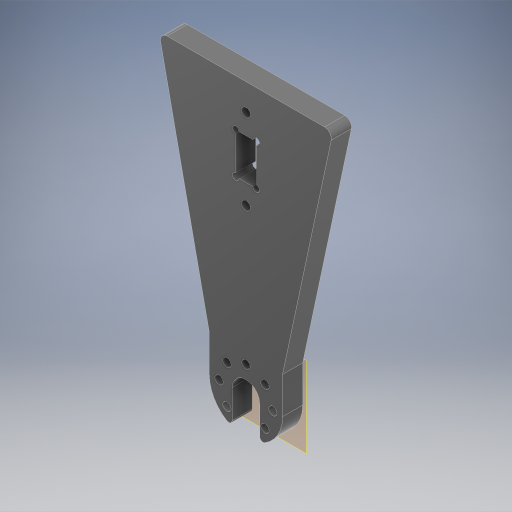
# Autodesk Inventor part: hand
Saved by Autodesk Inventor 2024 (Build 280153000, 153)
## iProperties
Created: 2024-09-04
Part Number: hand
Material: PMMA 플라스틱
Document SubType Name: Modeling
Designer: msi
Density: 1.188 g/cm^3
Appearance: 매끄러움 - 검은색
Mass: 19.7141 g
Surface Area: 78.213 cm^2
Volume: 16.5944 cm^3
Author: msi
Autodesk Inventor part; units mm, degrees
ref_plane "YZ Plane" through (0, 0, 0) normal (1, 0, 0) x (0, 1, 0)
ref_plane "XZ Plane" through (0, 0, 0) normal (0, 1, 0) x (-1, 0, 0)
ref_plane "XY Plane" through (0, 0, 0) normal (0, 0, 1) x (1, 0, 0)
ref_plane "작업 평면1" through (0, 0, 0) normal (0, 0, 1) x (1, 0, 0)
sketch "스케치1" plane through (0, 0, 0) normal (0, 0, 1) x (1, 0, 0)
  circle A0 centre (-5.6569, -5.6569) radius 1.2 projected
  circle A1 centre (5.6569, -5.6569) radius 1.2 projected
  circle A2 centre (5.6569, 5.6569) radius 1.2 projected
  circle A3 centre (-5.6569, 5.6569) radius 1.2 projected
  circle A4 centre (0, 0) radius 4 projected
  circle A5 centre (0, 0) radius 10.9 projected
  circle A6 centre (0, 8) radius 1.2 projected
  circle A7 centre (8, 0) radius 1.2 projected
  circle A8 centre (0, -8) radius 1.2 projected
  circle A9 centre (-8, 0) radius 1.2 projected
  line L0 (10.9, 0) -> (10.9, 10.9)
  line L1 (10.9, 10.9) -> (-10.9, 10.9)
  line L2 (-10.9, 10.9) -> (-10.9, 0)
  line L3 (-10.9, 10.9) -> (10.9, 10.9)
  line L4 (10.9, 80.9) -> (-10.9, 80.9)
  line L5 (10.9, 80.9) -> (25.9, 80.9)
  line L6 (25.9, 80.9) -> (10.9, 10.9)
  line L7 (-10.9, 80.9) -> (-25.9, 80.9)
  line L8 (-25.9, 80.9) -> (-10.9, 10.9)
  circle A10 centre (0, 72.9) radius 1.35
  circle A11 centre (0, 48.9) radius 1.35
  line L9 (-3.05, 54.85) -> (3.05, 54.85)
  line L10 (3.05, 54.85) -> (3.05, 66.95)
  line L11 (3.05, 66.95) -> (-3.05, 66.95)
  line L12 (-3.05, 66.95) -> (-3.05, 54.85)
  line L13 (-3.05, 54.85) -> (3.05, 66.95) construction
  line L14 (3.05, 54.85) -> (-3.05, 66.95) construction
  circle A12 centre (0, 0) radius 4.1
  circle A13 centre (5.6569, 5.6569) radius 1.25
  circle A14 centre (0, 8) radius 1.25
  circle A15 centre (-5.6569, 5.6569) radius 1.25
  circle A16 centre (-8, 0) radius 1.25
  circle A17 centre (-5.6569, -5.6569) radius 1.25
  circle A18 centre (0, -8) radius 1.25
  circle A19 centre (5.6569, -5.6569) radius 1.25
  circle A20 centre (8, 0) radius 1.25
  circle A21 centre (0, 0) radius 10.9
  line L15 (-4.1, 0) -> (-4.1, -10.0995)
  line L16 (4.1, 0) -> (4.1, -10.0995)
  point P0 (0, 0)
  point P1 (0, 60.9)
  dimension "d22" = 2.7
  dimension "d23" = 2.7
  dimension "d28" = 6.1
  dimension "d29" = 12.1
  dimension "d33" = 2.5
  dimension "d36" = 360
  constraints: 34 end point, 12 centre point, 6 point on circle, 4 parallel, 3 horizontal, 2 coincident, 2 midpoint, 1 concentric, 1 perpendicular, 1 point on line, 1 tangent, 1 vertical, 17 other
  measures "d22" diameter of A10
  measures "d23" diameter of A11
  measures "d28" distance of L11.end L10.end
  measures "d29" distance of L10.end L9.end
  measures "d33" diameter of A13
extrude "돌출6" add sketch "스케치1" along normal blind 6 contours A5 L16 A12 L15 | L2 L1 A5 | L1 L0 A5 | L1 L8 L7 L4 L5 L6 picked at (-5.5569, -1.7483)
fillet "모깎기2" radius 1 2 edges at (4.1, -10.0995, 3) (-4.1, -10.0995, 3)
fillet "모깎기3" radius 2 2 edges at (25.9, 80.9, 3) (-25.9, 80.9, 3)
sketch "스케치2" plane through (0, 0, 6) normal (0, 0, 1) x (1, 0, 0)
  line L0 (3.05, 66.95) -> (3.05, 54.85) projected
  line L1 (-3.05, 54.85) -> (-3.05, 66.95) projected
  line L2 (-3.05, 66.95) -> (3.05, 66.95) projected
  line L3 (3.05, 54.85) -> (-3.05, 54.85) projected
  circle A0 centre (3.05, 66.95) radius 1
  circle A1 centre (-3.05, 66.95) radius 1
  circle A2 centre (-3.05, 54.85) radius 1
  circle A3 centre (3.05, 54.85) radius 1
  point P0 (0, 0)
  dimension "d42" = 2
  dimension "d43" = 2
  dimension "d44" = 2
  dimension "d45" = 2
  constraints: 4 centre point, 4 coincident
  measures "d42" diameter of A0
  measures "d43" diameter of A1
  measures "d44" diameter of A2
  measures "d45" diameter of A3
extrude "돌출7" cut sketch "스케치2" against normal blind 10 contours L2 A0 L0 | L0 A0 L2 | A3 L3 L0 | L0 L3 A3 | A1 L1 L2 | L2 L1 A1 | A2 L1 L3 | L3 L1 A2
